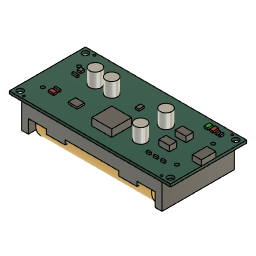
USB_UPS (Autodesk Fusion 360 archive; units mm, degrees)
design "MicroUSB_UPS"
Autodesk Fusion 360 part; units mm, degrees
sketch "pcb" plane through (0, 0, 0) normal (0, 0, 1) x (1, 0, 0)
  line L0 (-44.5, 21) -> (44.5, 21)
  line L1 (44.5, 21) -> (44.5, -21)
  line L2 (44.5, -21) -> (-44.5, -21)
  line L3 (-44.5, -21) -> (-44.5, 21)
  line L4 (-44.5, 21) -> (44.5, -21) construction
  line L5 (44.5, 21) -> (-44.5, -21) construction
  line L6 (-44.5, 21) -> (-41.5, 21) construction
  line L7 (-41.5, 21) -> (-41.5, 18) construction
  circle A0 centre (-41.5, 18) radius 1.7
  line L8 (0, 2.5) -> (0, 20)
  circle A1 centre (41.5, 18) radius 1.7
  line L9 (20, 0) -> (2.5, 0)
  circle A2 centre (-41.5, -18) radius 1.7
  circle A3 centre (41.5, -18) radius 1.7
  circle A4 centre (38, 19.5) radius 0.6
  circle A5 centre (-38, 19.5) radius 0.6
  circle A6 centre (-38, -19.5) radius 0.6
  circle A7 centre (38, -19.5) radius 0.6
  circle A8 centre (37, 10) radius 1
  circle A9 centre (-37, 10) radius 1
  circle A10 centre (-37, -10) radius 1
  circle A11 centre (37, -10) radius 1
  dimension "d1" = 89
  dimension "d2" = 42
  dimension "d3" = 3
  dimension "d4" = 3
  dimension "d5" = 3.4
  dimension "d12" = 1.2
  dimension "d13" = 2
  constraint horizontal L0
  constraint perpendicular L0 L1
  constraint parallel L0 L2
  constraint parallel L1 L3
  constraint coincident L4 origin
  constraint coincident L5 origin
  constraint perpendicular L3 L6
  constraint perpendicular L6 L7
  constraint coincident L7.end A0.centre
  constraint symmetric A0 L8 A1
  constraint symmetric A0 L9 A2
  constraint symmetric A1 L9 A3
  constraint symmetric L8 A4 A5
  constraint symmetric L9 A4 A7
  constraint symmetric L9 A5 A6
  constraint symmetric L8 A8 A9
  constraint symmetric L9 A9 A10
  constraint symmetric L9 A8 A11
  measures "d1" distance of L1.end L2.end
  measures "d2" distance of L0.end L1.end
  measures "d3" distance of L0.start L6.end
  measures "d4" distance of L6.end L7.end
  measures "d5" diameter of A0
  measures "d12" diameter of A4
  measures "d13" diameter of A8
sketch "components" plane through (0, 0, 0) normal (0, 0, 1) x (1, 0, 0)
  line L0 (44.5, -4) -> (39.5, -4)
  line L1 (39.5, -4) -> (39.5, 4)
  line L2 (39.5, 4) -> (44.5, 4)
  line L3 (44.5, 4) -> (44.5, -4)
  line L4 (44.5, -4) -> (39.5, 4) construction
  line L5 (39.5, -4) -> (44.5, 4) construction
  circle A0 centre (15, 6) radius 3.25
  circle A1 centre (-15, 6) radius 3.25
  circle A2 centre (-24, 6) radius 3.25
  line L6 (-1, 8) -> (1, 8)
  line L7 (1, 8) -> (1, 5)
  line L8 (1, 5) -> (-1, 5)
  line L9 (-1, 5) -> (-1, 8)
  line L10 (-5, -4) -> (6, -4)
  line L11 (6, -4) -> (6, -15)
  line L12 (6, -15) -> (-5, -15)
  line L13 (-5, -15) -> (-5, -4)
  circle A3 centre (15, -8) radius 3.25
  line L14 (23, 7) -> (29, 7)
  line L15 (29, 7) -> (29, 3)
  line L16 (29, 3) -> (23, 3)
  line L17 (23, 3) -> (23, 7)
  line L18 (23, -2) -> (28.8532, -2)
  line L19 (28.8532, -2) -> (28.8532, -6)
  line L20 (28.8532, -6) -> (23, -6)
  line L21 (23, -6) -> (23, -2)
  line L22 (30, 18) -> (32, 18)
  line L23 (32, 18) -> (32, 15)
  line L24 (32, 15) -> (30, 15)
  line L25 (30, 15) -> (30, 18)
  line L26 (29, 18) -> (27, 18)
  line L27 (27, 18) -> (27, 15)
  line L28 (27, 15) -> (29, 15)
  line L29 (29, 15) -> (29, 18)
  line L30 (33, 17) -> (34, 17)
  line L31 (34, 17) -> (34, 15)
  line L32 (34, 15) -> (33, 15)
  line L33 (33, 15) -> (33, 17)
  line L34 (35, 17) -> (36, 17)
  line L35 (36, 17) -> (36, 15)
  line L36 (36, 15) -> (35, 15)
  line L37 (35, 15) -> (35, 17)
  line L38 (-33, -9) -> (-30, -9)
  line L39 (-30, -9) -> (-30, -11)
  line L40 (-30, -11) -> (-33, -11)
  line L41 (-33, -11) -> (-33, -9)
  line L42 (-33, -7) -> (-30, -7)
  line L43 (-30, -7) -> (-30, -8)
  line L44 (-30, -8) -> (-33, -8)
  line L45 (-33, -8) -> (-33, -7)
  line L46 (-22, -7) -> (-17, -7)
  line L47 (-17, -7) -> (-17, -11)
  line L48 (-17, -11) -> (-22, -11)
  line L49 (-22, -11) -> (-22, -7)
  line L50 (-35, 9) -> (-33, 9)
  line L51 (-33, 9) -> (-33, 7)
  line L52 (-33, 7) -> (-35, 7)
  line L53 (-35, 7) -> (-35, 9)
  line L54 (-35, 5) -> (-32, 5)
  line L55 (-32, 5) -> (-32, 4)
  line L56 (-32, 4) -> (-35, 4)
  line L57 (-35, 4) -> (-35, 5)
  line L58 (23, -12) -> (25, -12)
  line L59 (25, -12) -> (25, -13)
  line L60 (25, -13) -> (23, -13)
  line L61 (23, -13) -> (23, -12)
  line L62 (27, -12) -> (29, -12)
  line L63 (29, -12) -> (29, -13)
  line L64 (29, -13) -> (27, -13)
  line L65 (27, -13) -> (27, -12)
  line L66 (31, -12) -> (33, -12)
  line L67 (33, -12) -> (33, -13)
  line L68 (33, -13) -> (31, -13)
  line L69 (31, -13) -> (31, -12)
  point P0 (42, 0)
  dimension "d6" = 5
  dimension "d7" = 8
  dimension "d8" = 6.5
  dimension "d9" = 6.5
  dimension "d10" = 6.5
  dimension "d11" = 6.5
  constraint horizontal L0
  constraint perpendicular L0 L1
  constraint parallel L0 L2
  constraint parallel L1 L3
  constraint coincident L4 P0
  constraint coincident L5 P0
  constraint horizontal L6
  constraint vertical L7
  constraint horizontal L8
  constraint vertical L9
  constraint horizontal L10
  constraint vertical L11
  constraint horizontal L12
  constraint vertical L13
  constraint horizontal L14
  constraint vertical L15
  constraint horizontal L16
  constraint vertical L17
  constraint horizontal L18
  constraint vertical L19
  constraint horizontal L20
  constraint vertical L21
  constraint horizontal L22
  constraint vertical L23
  constraint horizontal L24
  constraint vertical L25
  constraint horizontal L26
  constraint vertical L27
  constraint horizontal L28
  constraint vertical L29
  constraint horizontal L30
  constraint vertical L31
  constraint horizontal L32
  constraint vertical L33
  constraint horizontal L34
  constraint vertical L35
  constraint horizontal L36
  constraint vertical L37
  constraint horizontal L38
  constraint vertical L39
  constraint horizontal L40
  constraint vertical L41
  constraint horizontal L42
  constraint vertical L43
  constraint horizontal L44
  constraint vertical L45
  constraint horizontal L46
  constraint vertical L47
  constraint horizontal L48
  constraint vertical L49
  constraint horizontal L50
  constraint vertical L51
  constraint horizontal L52
  constraint vertical L53
  constraint horizontal L54
  constraint vertical L55
  constraint horizontal L56
  constraint vertical L57
  constraint horizontal L58
  constraint vertical L59
  constraint horizontal L60
  constraint vertical L61
  constraint horizontal L62
  constraint vertical L63
  constraint horizontal L64
  constraint vertical L65
  constraint horizontal L66
  constraint vertical L67
  constraint horizontal L68
  constraint vertical L69
  measures "d6" distance of L1.end L2.end
  measures "d7" distance of L0.end L1.end
  measures "d8" diameter of A0
  measures "d9" diameter of A1
  measures "d10" diameter of A2
  measures "d11" diameter of A3
ref_plane "WorkPlane1" through (0, 0, -1.5) normal (0, 0, 1) x (1, 0, 0)
sketch "plastic" plane through (0, 0, -1.5) normal (0, 0, 1) x (1, 0, 0)
  line L0 (38.75, 20) -> (-38.75, 20)
  line L1 (-38.75, 20) -> (-38.75, -20)
  line L2 (-38.75, -20) -> (38.75, -20)
  line L3 (38.75, -20) -> (38.75, 20)
  line L4 (38.75, 20) -> (-38.75, -20) construction
  line L5 (-38.75, 20) -> (38.75, -20) construction
  line L6 (35, -20) -> (35, 20)
  line L7 (38.75, -18) -> (-38.75, -18)
  line L8 (0, 1.75) -> (0, 22.5)
  line L9 (-35, -20) -> (-35, 20)
  line L10 (24.9665, -20) -> (24.9665, -18)
  line L11 (14.92, -20) -> (14.92, -18)
  line L12 (-25.0628, -20) -> (-25.0628, -18)
  line L13 (-14.7372, -20) -> (-14.7372, -18)
  line L14 (1.75, 0) -> (22.5, 0)
  line L15 (38.75, 18) -> (-38.75, 18)
  line L16 (-25.0628, 20) -> (-25.0628, 18)
  line L17 (-14.7372, 20) -> (-14.7372, 18)
  line L18 (14.92, 20) -> (14.92, 18)
  line L19 (24.9665, 20) -> (24.9665, 18)
  line L20 (35, -1) -> (-35, -1)
  line L21 (-35, -1) -> (-35, 1)
  line L22 (-35, 1) -> (35, 1)
  line L23 (35, 1) -> (35, -1)
  line L24 (35, -1) -> (-35, 1) construction
  line L25 (-35, -1) -> (35, 1) construction
  dimension "d15" = 77.5
  dimension "d16" = 40
  constraint horizontal L0
  constraint perpendicular L0 L1
  constraint parallel L0 L2
  constraint parallel L1 L3
  constraint coincident L4 origin
  constraint coincident L5 origin
  constraint coincident L0 L6.end
  constraint perpendicular L0 L6
  constraint coincident L2 L6.start
  constraint coincident L1 L7.end
  constraint perpendicular L1 L7
  constraint coincident L3 L7.start
  constraint symmetric L6.start L8 L9.start
  constraint symmetric L6.end L8 L9.end
  constraint coincident L2 L10.start
  constraint coincident L7 L10.end
  constraint perpendicular L7 L10
  constraint coincident L2 L11.start
  constraint coincident L7 L11.end
  constraint perpendicular L7 L11
  constraint coincident L2 L12.start
  constraint coincident L7 L12.end
  constraint perpendicular L7 L12
  constraint coincident L2 L13.start
  constraint coincident L7 L13.end
  constraint perpendicular L7 L13
  constraint symmetric L7.start L14 L15.start
  constraint symmetric L7.end L14 L15.end
  constraint symmetric L10.start L14 L19.start
  constraint symmetric L10.end L14 L19.end
  constraint symmetric L11.start L14 L18.start
  constraint symmetric L11.end L14 L18.end
  constraint symmetric L12.start L14 L16.start
  constraint symmetric L12.end L14 L16.end
  constraint symmetric L13.start L14 L17.start
  constraint symmetric L13.end L14 L17.end
  constraint horizontal L20
  constraint perpendicular L20 L21
  constraint parallel L20 L22
  constraint parallel L21 L23
  constraint coincident L24 origin
  constraint coincident L25 origin
  constraint coincident L6 L20.start
  measures "d15" distance of L1.end L2.end
  measures "d16" distance of L0.end L1.end
sketch "batteries" plane through (0, 0, 0) normal (1, 0, 0) x (0, 1, 0)
  circle A0 centre (10, -11) radius 9
  circle A1 centre (-10, -11) radius 9
  circle A2 centre (-10, -11) radius 3
  circle A3 centre (10, -11) radius 3
  dimension "d17" = 6
  dimension "d18" = 6
  constraint concentric A1 A2
  constraint concentric A0 A3
  measures "d17" diameter of A2
  measures "d18" diameter of A3
extrude "Extrude1" add sketch "components" along normal blind 8 contours A0 | A1 | A2 | A3 makes body 1 at (-11.754, 5.838, 5.3333) makes body 2 at (18.246, 5.838, 5.3333) makes body 3 at (-20.754, 5.838, 5.3333) makes body 4 at (18.246, -8.162, 5.3333)
extrude "Extrude2" add sketch "components" along normal blind 4 separate body contours L10 L11 L12 L13 makes body 5
extrude "Extrude3" add sketch "components" along normal blind 3 separate body contours L0 L1 L2 L3 | L14 L15 L16 L17 | L18 L19 L20 L21 makes body 6 at (41.1667, -1.3333, 0) makes body 7 at (25, 5.6667, 0) makes body 8 at (24.9511, -3.3333, 0)
extrude "Extrude4" add sketch "components" along normal blind 1 separate body contours L6 L7 L8 L9 | L22 L23 L24 L25 | L26 L27 L28 L29 | L30 L31 L32 L33 | L34 L35 L36 L37 | L38 L39 L40 L41 | L42 L43 L44 L45 | L46 L47 L48 L49 | L50 L51 L52 L53 | L54 L55 L56 L57 | L58 L59 L60 L61 | L62 L63 L64 L65 | L66 L67 L68 L69 makes body 9 at (23.6667, -12.3333, 0) makes body 10 at (27.6667, 17, 0) makes body 11 at (-34, 4.6667, 0) makes body 12 at (-32, -7.3333, 0) makes body 13 at (30.6667, 17, 0) makes body 14 at (27.6667, -12.3333, 0) makes body 15 at (35.3333, 16.3333, 0) makes body 16 at (-20.3333, -8.3333, 0) makes body 17 at (-34.3333, 8.3333, 0) makes body 18 at (-32, -9.6667, 0) makes body 19 at (33.3333, 16.3333, 0) makes body 20 at (-0.3333, 7, 0) makes body 21 at (31.6667, -12.3333, 0)
extrude "Extrude5" add sketch "pcb" against normal blind 1.5 separate body makes body 22
extrude "Extrude6" add sketch "plastic" against normal blind 10 separate body contours L0 L15 L18 L19 | L2 L7 L10 L11 | L0 L15 L16 L17 | L2 L7 L12 L13 makes body 23 at (-18.1791, 18, -4.8333) makes body 24 at (21.6177, 18, -8.1667) makes body 25 at (-21.621, -20, -8.1667) makes body 26 at (18.2688, -20, -8.1667)
extrude "Extrude7" add sketch "plastic" against normal blind 7.5 contours L0 L6 L15 L19 | L0 L8 L15 L18 | L2 L6 L7 L10 | L0 L8 L15 L17 | L0 L9 L15 L16 | L2 L7 L11 L13 | L2 L7 L9 L12 bodies 25 23 24 26
extrude "Extrude8" add sketch "plastic" against normal blind 15 contours L0 L3 L6 L15 | L3 L6 L7 L15 L23 | L2 L3 L6 L7 | L1 L7 L9 L15 L21 | L0 L1 L9 L15 | L1 L2 L7 L9 bodies 25 23
extrude "Extrude9" add sketch "batteries" along normal blind 33 and the other way blind 34 separate body contours A2 | A3 makes body 27 at (-22.6667, 12.9963, -11.1495) makes body 28 at (-22.6667, -7.0037, -11.1495)
extrude "Extrude10" add sketch "batteries" along normal blind 32 and the other way blind 32 separate body makes body 29 at (21.3333, 18.9888, -11.4486) makes body 30 at (21.3333, -1.0112, -11.4486)
named bodies: "pcb", "plastic", "bat_core1", "bat_core2", "bat1", "bat2"
